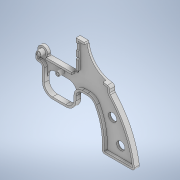
# Autodesk Inventor part: Telo_Desno_3
Saved by Autodesk Inventor 2021 (Build 250183000, 183)
## iProperties
Created: 2022-03-07
Part Number: Telo_Desno_3
Material: Generic
Document SubType Name: Modeling
Designer: Carlos Montoya
Density: 1 g/cm^3
Appearance: Default
Author: Carlos Montoya
Autodesk Inventor part; units mm, degrees
ref_plane "YZ Plane" through (0, 0, 0) normal (1, 0, 0) x (0, 1, 0)
ref_plane "XZ Plane" through (0, 0, 0) normal (0, 1, 0) x (-1, 0, 0)
sketch "Sketch1" plane through (0, 0, 0) normal (0, 0, 1) x (1, 0, 0)
  arc A0 (-24.5843, 100) -> (-1.6853, 72.55) centre (6.3147, 102.5) ccw
  arc A1 (-24.6853, 102.5) -> (-24.5843, 100) centre (6.3147, 102.5) ccw
  line L0 (-34.6853, 102.5) -> (-24.6853, 102.5)
  line L1 (-34.6853, 102.5) -> (-34.6853, 97.5)
  line L2 (-34.6853, 97.5) -> (-34.6853, 89.5)
  line L3 (-34.6853, 89.5) -> (-34.6853, 83)
  line L4 (-34.6853, 83) -> (-34.6853, 80)
  line L5 (-34.6853, 80) -> (-34.6853, 68.5)
  line L6 (-34.6853, 68.5) -> (-34.6853, 65.5)
  arc A2 (-36.6853, 63.5) -> (-34.6853, 65.5) centre (-36.6853, 65.5) ccw
  line L7 (-36.6853, 63.5) -> (-39.6853, 63.5)
  line L8 (-39.6853, 63.5) -> (-70.6853, 63.5)
  arc A3 (-71.6853, 64.5) -> (-70.9653, 63.54) centre (-70.6853, 64.5) ccw
  line L9 (-71.6853, 64.5) -> (-71.6853, 65.5)
  arc A4 (-70.9653, 63.54) -> (-70.6853, 63.5) centre (-70.6853, 64.5) ccw
  arc A5 (-71.6853, 65.5) -> (-83.6853, 65.5) centre (-77.6853, 65.5) ccw
  line L10 (-83.6853, 65.5) -> (-83.6853, 61.8944)
  line L11 (-83.6853, 61.8944) -> (-83.6853, 57.5)
  arc A6 (-83.6853, 57.5) -> (-80.6853, 54.5) centre (-80.6853, 57.5) ccw
  line L12 (-80.6853, 54.5) -> (-78.6853, 54.5)
  arc A7 (-75.6853, 51.5) -> (-78.6853, 54.5) centre (-78.6853, 51.5) ccw
  line L13 (-75.6853, 51.5) -> (-75.6853, 36)
  arc A8 (-75.6853, 36) -> (-63.1853, 23.5) centre (-63.1853, 36) ccw
  line L14 (-63.1853, 23.5) -> (-47.1853, 23.5)
  arc A9 (-47.1853, 23.5) -> (-34.6853, 36) centre (-47.1853, 36) ccw
  line L15 (-34.6853, 36) -> (-34.6853, 41)
  arc A10 (-27.1853, 48.5) -> (-34.6853, 41) centre (-27.1853, 41) ccw
  line L16 (-27.1853, 48.5) -> (-20.5538, 48.5)
  arc A11 (-11.7644, 43.2692) -> (-20.5538, 48.5) centre (-20.5538, 38.5) ccw
  arc A12 (-2.9879, 0.7692) -> (-11.7644, 43.2692) centre (-77.6853, 7.5) ccw
  arc A13 (-2.9879, 0.7692) -> (0, -2.5) centre (0, 0.5) ccw
  line L17 (0, -2.5) -> (33.3057, -2.5)
  arc A14 (33.3057, -2.5) -> (36.2787, 0.9018) centre (33.3057, 0.5) ccw
  arc A15 (36.2787, 0.9018) -> (7.1029, 63.1915) centre (-77.6853, -14.5) ccw
  arc A16 (6.3147, 65.2183) -> (7.1029, 63.1915) centre (9.3147, 65.2183) ccw
  line L18 (6.3147, 68.6326) -> (6.3147, 65.2183)
  arc A17 (6.3147, 68.6326) -> (3.5794, 71.6209) centre (3.3147, 68.6326) ccw
  arc A18 (-1.6853, 72.55) -> (3.5794, 71.6209) centre (6.3147, 102.5) ccw
  circle A19 centre (6.3147, 37.5) radius 5
  circle A20 centre (16.3147, 12.5) radius 5
  line L19 (-73.1853, 36) -> (-73.1853, 41)
  arc A21 (-63.1853, 51) -> (-73.1853, 41) centre (-63.1853, 41) ccw
  line L20 (-47.1853, 51) -> (-63.1853, 51)
  arc A22 (-37.1853, 41) -> (-47.1853, 51) centre (-47.1853, 41) ccw
  line L21 (-37.1853, 36) -> (-37.1853, 41)
  arc A23 (-47.1853, 26) -> (-37.1853, 36) centre (-47.1853, 36) ccw
  line L22 (-63.1853, 26) -> (-47.1853, 26)
  arc A24 (-73.1853, 36) -> (-63.1853, 26) centre (-63.1853, 36) ccw
  point P0 (0, 0)
  constraints: 46 end point, 46 point on circle, 25 centre point
extrude "Extrusion1" add sketch "Sketch1" along normal blind 2.5
sketch "Sketch2" plane through (0, 0, 2.5) normal (0, 0, 1) x (1, 0, 0)
  arc A0 (-24.5843, 100) -> (-1.6853, 72.55) centre (6.3147, 102.5) ccw
  arc A1 (-24.6853, 102.5) -> (-24.5843, 100) centre (6.3147, 102.5) ccw
  line L0 (-34.6853, 102.5) -> (-24.6853, 102.5)
  line L1 (-34.6853, 102.5) -> (-34.6853, 97.5)
  line L2 (-34.6853, 97.5) -> (-34.6853, 89.5)
  line L3 (-34.6853, 89.5) -> (-34.6853, 83)
  line L4 (-34.6853, 83) -> (-34.6853, 80)
  line L5 (-34.6853, 80) -> (-34.6853, 68.5)
  line L6 (-34.6853, 68.5) -> (-34.6853, 65.5)
  arc A2 (-36.6853, 63.5) -> (-34.6853, 65.5) centre (-36.6853, 65.5) ccw
  line L7 (-36.6853, 63.5) -> (-39.6853, 63.5)
  line L8 (-39.6853, 63.5) -> (-70.6853, 63.5)
  arc A3 (-71.6853, 64.5) -> (-70.9653, 63.54) centre (-70.6853, 64.5) ccw
  line L9 (-71.6853, 64.5) -> (-71.6853, 65.5)
  arc A4 (-70.9653, 63.54) -> (-70.6853, 63.5) centre (-70.6853, 64.5) ccw
  arc A5 (-71.6853, 65.5) -> (-83.6853, 65.5) centre (-77.6853, 65.5) ccw
  line L10 (-83.6853, 65.5) -> (-83.6853, 61.8944)
  line L11 (-83.6853, 61.8944) -> (-83.6853, 57.5)
  arc A6 (-83.6853, 57.5) -> (-80.6853, 54.5) centre (-80.6853, 57.5) ccw
  line L12 (-80.6853, 54.5) -> (-78.6853, 54.5)
  arc A7 (-75.6853, 51.5) -> (-78.6853, 54.5) centre (-78.6853, 51.5) ccw
  line L13 (-75.6853, 51.5) -> (-75.6853, 36)
  arc A8 (-75.6853, 36) -> (-63.1853, 23.5) centre (-63.1853, 36) ccw
  line L14 (-63.1853, 23.5) -> (-47.1853, 23.5)
  arc A9 (-47.1853, 23.5) -> (-34.6853, 36) centre (-47.1853, 36) ccw
  line L15 (-34.6853, 36) -> (-34.6853, 41)
  arc A10 (-27.1853, 48.5) -> (-34.6853, 41) centre (-27.1853, 41) ccw
  line L16 (-27.1853, 48.5) -> (-20.5538, 48.5)
  arc A11 (-11.7644, 43.2692) -> (-20.5538, 48.5) centre (-20.5538, 38.5) ccw
  arc A12 (-2.9879, 0.7692) -> (-11.7644, 43.2692) centre (-77.6853, 7.5) ccw
  arc A13 (-2.9879, 0.7692) -> (0, -2.5) centre (0, 0.5) ccw
  line L17 (0, -2.5) -> (33.3057, -2.5)
  arc A14 (33.3057, -2.5) -> (36.2787, 0.9018) centre (33.3057, 0.5) ccw
  arc A15 (36.2787, 0.9018) -> (7.1029, 63.1915) centre (-77.6853, -14.5) ccw
  arc A16 (6.3147, 65.2183) -> (7.1029, 63.1915) centre (9.3147, 65.2183) ccw
  line L18 (6.3147, 68.6326) -> (6.3147, 65.2183)
  arc A17 (6.3147, 68.6326) -> (3.5794, 71.6209) centre (3.3147, 68.6326) ccw
  arc A18 (-1.6853, 72.55) -> (3.5794, 71.6209) centre (6.3147, 102.5) ccw
  circle A19 centre (6.3147, 37.5) radius 5
  circle A20 centre (16.3147, 12.5) radius 5
  line L19 (-73.1853, 36) -> (-73.1853, 41)
  arc A21 (-63.1853, 51) -> (-73.1853, 41) centre (-63.1853, 41) ccw
  line L20 (-47.1853, 51) -> (-63.1853, 51)
  arc A22 (-37.1853, 41) -> (-47.1853, 51) centre (-47.1853, 41) ccw
  line L21 (-37.1853, 36) -> (-37.1853, 41)
  arc A23 (-47.1853, 26) -> (-37.1853, 36) centre (-47.1853, 36) ccw
  line L22 (-63.1853, 26) -> (-47.1853, 26)
  arc A24 (-73.1853, 36) -> (-63.1853, 26) centre (-63.1853, 36) ccw
  line L23 (-73.1853, 51.5) -> (-73.1853, 36)
  arc A25 (-73.1853, 51.5) -> (-78.6853, 57) centre (-78.6853, 51.5) ccw
  line L24 (-80.6853, 57) -> (-78.6853, 57)
  arc A26 (-81.1853, 57.5) -> (-80.6853, 57) centre (-80.6853, 57.5) ccw
  line L25 (-81.1853, 59.4378) -> (-81.1853, 57.5)
  arc A27 (-83.6853, 61.8944) -> (-81.1853, 59.4378) centre (-77.6853, 65.5) ccw
  arc A28 (-83.6853, 61.8944) -> (-81.1853, 59.4378) centre (-77.6853, 65.5) ccw
  circle A29 centre (-77.6853, 65.5) radius 3
  line L26 (-39.6853, 61) -> (-70.6853, 61)
  arc A30 (-72.0897, 61.2941) -> (-70.9653, 63.54) centre (-77.6853, 65.5) ccw
  line L27 (-39.6853, 63.5) -> (-39.6853, 61)
  arc A31 (-72.0897, 61.2941) -> (-70.9653, 63.54) centre (-77.6853, 65.5) ccw
  line L28 (-32.1853, 68.5) -> (-34.6853, 68.5)
  line L29 (-32.1853, 80) -> (-32.1853, 68.5)
  line L30 (-32.1853, 89.5) -> (-32.1853, 83)
  line L31 (-32.1853, 80) -> (-32.1853, 83)
  line L32 (-32.1853, 89.5) -> (-34.6853, 89.5)
  line L33 (-32.1853, 97.5) -> (-34.6853, 97.5)
  line L34 (-32.1853, 100) -> (-32.1853, 97.5)
  line L35 (-24.5843, 100) -> (-32.1853, 100)
  arc A32 (-27.1853, 51) -> (-37.1853, 41) centre (-27.1853, 41) ccw
  line L36 (-27.1853, 51) -> (-20.5538, 51)
  arc A33 (-9.567, 44.4615) -> (-20.5538, 51) centre (-20.5538, 38.5) ccw
  arc A34 (-0.498, 0.5449) -> (-9.567, 44.4615) centre (-77.6853, 7.5) ccw
  line L37 (0, 0) -> (33.3057, 0)
  arc A35 (-0.498, 0.5449) -> (0, 0) centre (0, 0.5) ccw
  arc A36 (33.3057, 0) -> (33.8012, 0.567) centre (33.3057, 0.5) ccw
  arc A37 (33.8012, 0.567) -> (5.2597, 61.5026) centre (-77.6853, -14.5) ccw
  line L38 (3.8147, 65.2183) -> (3.8147, 68.6326)
  arc A38 (3.8147, 65.2183) -> (5.2597, 61.5026) centre (9.3147, 65.2183) ccw
  arc A39 (3.8147, 68.6326) -> (3.3589, 69.1307) centre (3.3147, 68.6326) ccw
  arc A40 (-1.6853, 69.9692) -> (3.3589, 69.1307) centre (6.3147, 102.5) ccw
  line L39 (-1.6853, 69.9692) -> (-1.6853, 72.55)
  circle A41 centre (-54.6853, 55.5) radius 2.5
  circle A42 centre (-54.6853, 55.5) radius 1.25
  circle A43 centre (-77.6853, 65.5) radius 1.5
  arc A44 (-74.1853, 64.5) -> (-70.6853, 61) centre (-70.6853, 64.5) ccw
  constraints: 80 end point, 78 point on circle, 45 centre point
extrude "Extrusion2" add sketch "Sketch2" along normal blind 3.5 contours L35 L34 L33 L1 L0 A1 | A18 A17 L18 A16 A15 A14 L17 A13 A12 A11 L16 A10 L15 A9 L14 A8 L13 A7 L12 A6 L11 A27 L25 A26 L24 A25 L23 L19 A24 L22 A23 L21 A32 L36 A33 A34 A35 L37 A36 A37 A38 L38 A39 A40 L39 | L32 L30 L31 L29 L28 L5 L4 L3 | L27 L26 A44 A30 A4 L8 | A29 | A41
sketch "Sketch3" plane through (0, 0, 2.5) normal (0, 0, 1) x (1, 0, 0)
  line L0 (-83.6853, 65.5) -> (-83.6853, 61.8944)
  arc A0 (-83.6853, 61.8944) -> (-81.1853, 59.4378) centre (-77.6853, 65.5) ccw
  arc A1 (-71.6853, 65.5) -> (-83.6853, 65.5) centre (-77.6853, 65.5) ccw
  line L1 (-71.6853, 64.5) -> (-71.6853, 65.5)
  arc A2 (-71.6853, 64.5) -> (-70.9653, 63.54) centre (-70.6853, 64.5) ccw
  arc A3 (-72.0897, 61.2941) -> (-70.9653, 63.54) centre (-77.6853, 65.5) ccw
  arc A4 (-74.1853, 64.5) -> (-72.0897, 61.2941) centre (-70.6853, 64.5) ccw
  line L2 (-74.1853, 65.5) -> (-74.1853, 64.5)
  arc A5 (-74.1853, 65.5) -> (-81.1853, 65.5) centre (-77.6853, 65.5) ccw
  line L3 (-81.1853, 59.4378) -> (-81.1853, 65.5)
  point P0 (0, 0)
  constraints: 12 point on circle, 8 end point, 6 centre point
extrude "Extrusion3" add sketch "Sketch3" along normal blind 1
sketch "Sketch4" plane through (0, 0, 2.5) normal (0, 0, 1) x (1, 0, 0)
  line L0 (-34.6853, 97.5) -> (-34.6853, 89.5)
  line L1 (-32.1853, 89.5) -> (-34.6853, 89.5)
  line L2 (-32.1853, 89.5) -> (-32.1853, 97.5)
  line L3 (-32.1853, 97.5) -> (-34.6853, 97.5)
  point P0 (0, 0)
  constraints: 8 end point
extrude "Extrusion4" add sketch "Sketch4" along normal blind 2
sketch "Sketch6" plane through (-75.6853, 36, 0) normal (-1, 0, 0) x (0, 0, 1)
  line L0 (6, 66.5) -> (1, 66.5)
  line L1 (6, 66.5) -> (6, 61.5)
  line L2 (6, 61.5) -> (4.5, 61.5)
  line L3 (4.5, 61.5) -> (4.5, 53.5)
  line L4 (4.5, 53.5) -> (6, 53.5)
  line L5 (6, 53.5) -> (6, 47)
  arc A0 (6, 47) -> (6, 44) centre (6, 45.5) ccw
  line L6 (6, 44) -> (6, 32.5)
  line L7 (2.5, 32.5) -> (6, 32.5)
  line L8 (0, 63) -> (0, 58.7004)
  line L9 (1, 63) -> (1, 66.5)
  line L10 (0, 63) -> (1, 63)
  line L11 (0, 63) -> (0, 66.5)
  line L12 (0, 66.5) -> (1, 66.5)
  line L13 (6, 47) -> (6, 44)
  line L14 (0, 66.5) -> (0, 29.5) projected
  point P0 (0, -36)
  constraints: 28 end point, 2 point on circle, 1 centre point, 1 parallel, 1 perpendicular, 1 vertical
extrude "Extrusion5" cut sketch "Sketch6" against normal blind 57.5625
sketch "Sketch7" plane through (-77.6853, 65.5, 6) normal (0, 0, 1) x (1, 0, 0)
  circle A0 centre (0, 0) radius 1.5 projected
  circle A1 centre (0, 0) radius 3
  circle A2 centre (23, -10) radius 1.25 projected
  circle A3 centre (23, -10) radius 2.524
  point P0 (77.6853, -65.5)
  constraints: 2 centre point, 2 coincident
extrude "Extrusion6" add sketch "Sketch7" along normal blind 2.5 and the other way blind 4
fillet "Fillet1" radius 0.5 1 edges at (-79.1853, 65.5, 8.5)
fillet "Fillet2" radius 0.5 1 edges at (-55.9353, 55.5, 8.5)
ref_plane "Work Plane1" through (-70.6853, 81.5, 0) normal (0, 1, 0) x (1, 0, 0)
sketch "Sketch11" plane through (-70.6853, 81.5, 0) normal (0, 1, 0) x (1, 0, 0)
  arc A0 (0.7921, 14.2204) -> (7.0973, 5.7204) centre (-9.8732, -0.2796) ccw
  line L0 (0.1268, 5.7204) -> (0.1268, 14.2204)
  line L1 (0.7921, 5.7204) -> (0.7921, 14.2204)
  line L2 (0.1268, 14.2204) -> (0.7921, 14.2204)
  line L3 (0.7921, 5.7204) -> (0.1268, 5.7204)
  line L4 (0.7921, 5.7204) -> (7.0973, 5.7204)
  line L5 (36, 0) -> (36, -6) projected
  line L6 (36, 0) -> (26, 0)
  line L7 (23.5, 0) -> (36, 0) projected
  line L8 (26, 0) -> (26, 14.5)
  line L9 (43.5, -6) -> (36, -6) projected
  line L10 (36, -6) -> (26, -6)
  circle A1 centre (26, -6) radius 18
  line L11 (36, 0) -> (36.665, 0)
  line L12 (36.665, 0) -> (36.665, 14.5)
  line L13 (36, 0) -> (36, 14.5)
  line L14 (36.665, 0) -> (9.0294, 0)
  line L15 (36, 0) -> (36, -2.5) projected
  line L16 (42.9706, 0) -> (36.665, 0)
  point P0 (70.6853, 0)
  point P1 (0, 4.5)
  point P2 (26, 12)
  dimension "d23" = 10
  dimension "d24" = 14.5
  dimension "d25" = 10
  dimension "d26" = 36
  dimension "d27" = 0.665
  dimension "d28" = 14.5
  constraints: 26 end point, 4 horizontal, 4 point on circle, 3 perpendicular, 2 centre point, 1 coincident, 1 point on line, 1 vertical, 4 other
  measures "d23" distance of L5.start L6.end
  measures "d24" distance of L6.end L8.end
  measures "d25" distance of L5.end L10.end
  measures "d26" diameter of A1
  measures "d27" distance of L5.start L11.end
  measures "d28" distance of L11.end L12.end
revolve "Revolution1" add sketch "Sketch11" angle 180 mid plane about axis through (-44.6853, 81.5, 0) along (0, 0, -1) contours L13 A1 L12 L11 | L6 L8 A1 L13 | L12 A1 L16
sketch "Sketch12" plane through (-70.6853, 81.5, 0) normal (0, 1, 0) x (1, 0, 0)
  arc A0 (0.7921, 14.2204) -> (7.0973, 5.7204) centre (-9.8732, -0.2796) ccw
  line L0 (0.1268, 5.7204) -> (0.1268, 14.2204)
  line L1 (0.7921, 5.7204) -> (0.7921, 14.2204)
  line L2 (0.1268, 14.2204) -> (0.7921, 14.2204)
  line L3 (0.7921, 5.7204) -> (0.1268, 5.7204)
  line L4 (0.7921, 5.7204) -> (7.0973, 5.7204)
  line L5 (36, 0) -> (36, -6)
  line L6 (36, 0) -> (26, 0)
  line L7 (23.5, 0) -> (36, 0)
  line L8 (26, 0) -> (26, 14.5)
  line L9 (43.5, -6) -> (36, -6)
  line L10 (36, -6) -> (26, -6)
  circle A1 centre (26, -6) radius 18
  line L11 (36, 0) -> (36.665, 0)
  line L12 (36.665, 0) -> (36.665, 14.5)
  line L13 (36, 0) -> (36, 14.5)
  line L14 (36.665, 0) -> (9.0294, 0)
  line L15 (36, 0) -> (36, -2.5)
  line L16 (42.9706, 0) -> (36.665, 0)
  arc A2 (42.9706, 0) -> (26, 12) centre (26, -6) ccw projected
  line L17 (36.665, 8.5003) -> (36.665, 0)
  line L18 (36.665, 0) -> (20.1181, 0)
  line L19 (20.1181, 0) -> (20.1181, 13.2816)
  line L20 (20.1181, 13.2816) -> (36.665, 13.2816)
  line L21 (36.665, 13.2816) -> (36.665, 0)
  point P0 (70.6853, 0)
  point P1 (70.6853, 0)
  point P2 (0, 4.5)
  point P3 (26, 12)
  point P4 (20.1181, 11.0119)
  point P5 (26, 12)
  dimension "d30" = 10
  dimension "d31" = 14.5
  dimension "d32" = 10
  dimension "d33" = 36
  dimension "d34" = 0.665
  dimension "d35" = 14.5
  constraints: 44 end point, 5 horizontal, 5 point on circle, 4 perpendicular, 2 centre point, 2 parallel, 2 point on line, 1 coincident, 1 collinear, 1 vertical, 4 other
  measures "d30" distance of L5.start L6.end
  measures "d31" distance of L6.end L8.end
  measures "d32" distance of L5.end L10.end
  measures "d33" diameter of A1
  measures "d34" distance of L5.start L11.end
  measures "d35" distance of L11.end L12.end
extrude "Extrusion7" cut sketch "Sketch12" against normal mid plane 48.1 contours L13 A1 L12 L11 | L6 L8 A1 L13 | L13 L20 L12 A1 | A1 L8 L20 L13 | A1 L19 L20 L8
sketch "Sketch13" plane through (-34.0203, 81.5, 6) normal (-1, 0, 0) x (0, 0, 1)
  arc A0 (-6, 13.2007) -> (-6, -13.2007) centre (0, 0) ccw projected
  line L0 (-6, -13.2007) -> (-6, 13.2007) projected
  point P0 (-6, -81.5)
extrude "Extrusion8" add sketch "Sketch13" along normal blind 0.665
body "Solid1"
